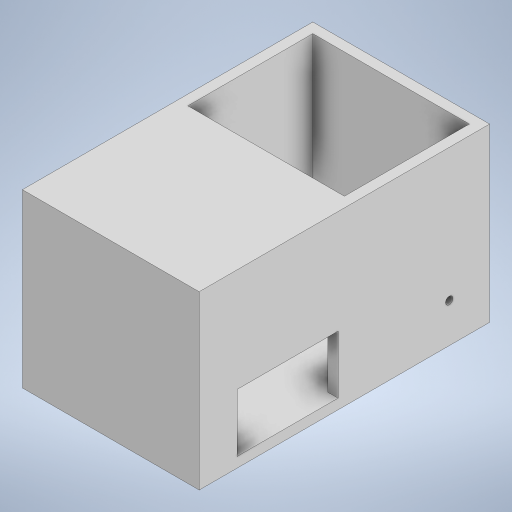
# Autodesk Inventor part: самосвал кузов
Saved by Autodesk Inventor 2023.2 (Build 272271000, 271)
## iProperties
Created: 2024-01-18
Part Number: самосвал кузов
Material: Типовые
Document SubType Name: Modeling
Designer: парпа
Density: 1 g/cm^3
Appearance: По умолчанию
Author: парпа
Autodesk Inventor part; units mm, degrees
ref_plane "YZ Plane" through (0, 0, 0) normal (1, 0, 0) x (0, 1, 0)
ref_plane "XZ Plane" through (0, 0, 0) normal (0, 1, 0) x (-1, 0, 0)
ref_plane "XY Plane" through (0, 0, 0) normal (0, 0, 1) x (1, 0, 0)
sketch "Эскиз1" plane through (0, 0, 0) normal (0, 1, 0) x (-1, 0, 0)
  line L0 (-35, 57.5) -> (35, 57.5)
  line L1 (35, 57.5) -> (35, -57.5)
  line L2 (35, -57.5) -> (-35, -57.5)
  line L3 (-35, -57.5) -> (-35, 57.5)
  line L4 (-35, 57.5) -> (35, -57.5) construction
  line L5 (35, 57.5) -> (-35, -57.5) construction
  point P0 (0, 0)
  dimension "d0" = 115
  dimension "d1" = 70
  constraints: 12 end point, 2 midpoint, 2 parallel, 1 horizontal, 1 perpendicular
  measures "d0" distance of L0.end L1.end
  measures "d1" distance of L0.start L0.end
extrude "Выдавливание1" add sketch "Эскиз1" along normal blind 4
sketch "Эскиз2" plane through (0, 4, 0) normal (0, 1, 0) x (1, 0, 0)
  line L0 (35, 57.5) -> (-35, 57.5) projected
  line L1 (35, -57.5) -> (-35, -57.5)
  line L2 (-35, -57.5) -> (-35, 57.5)
  line L3 (-35, 57.5) -> (35, 57.5)
  line L4 (35, 57.5) -> (35, -57.5)
  line L5 (35, -57.5) -> (-35, 57.5) construction
  line L6 (-35, -57.5) -> (35, 57.5) construction
  line L7 (31, -53.5) -> (-31, -53.5)
  line L8 (-31, -53.5) -> (-31, 53.5)
  line L9 (-31, 53.5) -> (31, 53.5)
  line L10 (31, 53.5) -> (31, -53.5)
  line L11 (31, -53.5) -> (-31, 53.5) construction
  line L12 (-31, -53.5) -> (31, 53.5) construction
  point P0 (0, 0)
  dimension "d4" = 4
  dimension "d5" = 4
  constraints: 24 end point, 4 midpoint, 4 parallel, 2 horizontal, 2 perpendicular
  measures "d4" distance between parallel lines of L2 L8
  measures "d5" distance between parallel lines of L7 L1
extrude "Выдавливание2" add sketch "Эскиз2" along normal blind 64
sketch "Эскиз3" plane through (35, 0, 57.5) normal (1, 0, 0) x (0, 0, -1)
  line L0 (111, 4) -> (4, 4) projected
  line L1 (15, 4) -> (55, 4)
  line L2 (55, 4) -> (55, 27)
  line L3 (55, 27) -> (15, 27)
  line L4 (15, 27) -> (15, 4)
  point P0 (57.5, 0)
  point P1 (0, 0)
  dimension "d9" = 40
  dimension "d10" = 23
  constraints: 8 end point, 2 parallel, 1 horizontal, 1 perpendicular, 1 point on line
  measures "d9" distance of L2.end L3.end
  measures "d10" distance of L1.end L2.end
extrude "Выдавливание3" cut sketch "Эскиз3" against normal blind 75
sketch "Эскиз4" plane through (35, 0, 57.5) normal (1, 0, 0) x (0, 0, -1)
  line L0 (55, 27) -> (55, 4) projected
  circle A0 centre (99, 15.5) radius 1.5
  point P0 (57.5, 0)
  dimension "d14" = 3
  constraints: 1 centre point
  measures "d14" diameter of A0
extrude "Выдавливание4" cut sketch "Эскиз4" against normal blind 75
sketch "Эскиз5" plane through (-31, 4, -53.5) normal (1, 0, 0) x (0, 0, -1)
  line L0 (-107, 0) -> (-107, 64) projected
  line L1 (-107, 64) -> (-49.5, 64)
  line L2 (-49.5, 64) -> (-49.5, 35.4088)
  line L3 (-49.5, 35.4088) -> (-53.5, 35.4088)
  line L4 (-53.5, 35.4088) -> (-53.5, 60)
  line L5 (-53.5, 60) -> (-107, 60)
  line L6 (-107, 60) -> (-107, 64)
  point P0 (-53.5, -4)
  dimension "d17" = 4
  dimension "d18" = 4
  constraints: 12 end point, 5 perpendicular, 1 horizontal
  measures "d17" distance between parallel lines of L5 L1
  measures "d18" distance between parallel lines of L4 L2
extrude "Выдавливание5" add sketch "Эскиз5" along normal blind 62
sketch "Эскиз6" plane through (0, 0, 0) normal (0, -1, 0) x (1, 0, 0)
  line L0 (-20.5745, 51.4953) -> (20.4255, 51.4953)
  line L1 (20.4255, 51.4953) -> (20.4255, 46.4953)
  line L2 (20.4255, 46.4953) -> (-20.5745, 46.4953)
  line L3 (-20.5745, 46.4953) -> (-20.5745, 51.4953)
  line L4 (-20.5745, 51.4953) -> (20.4255, 46.4953) construction
  line L5 (20.4255, 51.4953) -> (-20.5745, 46.4953) construction
  point P0 (0, 0)
  point P1 (-0.0745, 48.9953)
  dimension "d21" = 5
  dimension "d22" = 41
  constraints: 12 end point, 2 midpoint, 2 parallel, 1 horizontal, 1 perpendicular
  measures "d21" distance of L0.end L1.end
  measures "d22" distance of L1.end L2.end
extrude "Выдавливание6" cut sketch "Эскиз6" against normal blind 10
